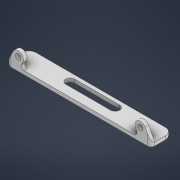
# Autodesk Inventor part: PCB Mount Support
Saved by Autodesk Inventor 2022.1 (Build 261234000, 234)
## iProperties
Created: 2022-01-06
Part Number: PCB Mount Support
Material: Generic
Document SubType Name: Modeling
Designer: Santiago Martínez
Mass: 1.78141 g
Surface Area: 23.5704 cm^2
Volume: 1.78141 cm^3
Density: 1 g/cm^3
Appearance: Default
Author: Santiago Martínez
Autodesk Inventor part; units mm, degrees
ref_plane "YZ Plane" through (0, 0, 0) normal (1, 0, 0) x (0, 1, 0)
ref_plane "XZ Plane" through (0, 0, 0) normal (0, 1, 0) x (-1, 0, 0)
ref_plane "XY Plane" through (0, 0, 0) normal (0, 0, 1) x (1, 0, 0)
sketch "Sketch1" plane through (0, 0, 0) normal (0, 1, 0) x (-1, 0, 0)
  line L0 (-27.5, -7.5) -> (-52.5, -7.5) construction
  line L1 (-27.5, -5) -> (-52.5, -5)
  line L2 (-52.5, -10) -> (-27.5, -10)
  arc A0 (-27.5, -10) -> (-27.5, -5) centre (-27.5, -7.5) ccw
  arc A1 (-52.5, -5) -> (-52.5, -10) centre (-52.5, -7.5) ccw
  line L3 (-4, -12) -> (-76, -12)
  line L4 (-80, -8) -> (-80, 0)
  line L5 (-80, 0) -> (0, 0)
  line L6 (0, 0) -> (0, -8)
  arc A2 (-4, -12) -> (0, -8) centre (-4, -8) ccw
  arc A3 (-80, -8) -> (-76, -12) centre (-76, -8) ccw
  point P0 (-40, -7.5)
  point P1 (-80, -12)
  point P2 (-40, -12)
  dimension "d0" = 25
  dimension "d1" = 5
  dimension "d2" = 80
  dimension "d3" = 12
  dimension "d5" = 4
  dimension "d6" = 2
  constraints: 16 end point, 8 point on circle, 8 tangent, 4 centre point, 3 parallel, 2 horizontal, 2 midpoint, 2 point on line, 1 coincident, 1 equal radius, 1 perpendicular, 1 vertical alignment
  measures "d0" distance of L0.start L0.end
  measures "d1" diameter of A1
  measures "d2" distance of L4.end L5.end
  measures "d3" distance of point (-80, -12) L4.end
  measures "d5" radius of A2
  measures "d6" distance between parallel lines of L2 L3
extrude "Extrusion1" add sketch "Sketch1" along normal blind 2
sketch "Sketch2" plane through (0, 0, 0) normal (0, 0, 1) x (1, 0, 0)
  circle A0 centre (6, 7) radius 1.5
  circle A1 centre (74, 7) radius 1.5
  line L0 (0, 0) -> (0, 2) projected
  line L1 (80, 0) -> (80, 2) projected
  line L2 (0, 2) -> (80, 2) projected
  line L3 (4, 2) -> (0, 2) projected
  line L4 (76, 2) -> (4, 2) projected
  line L5 (9.2479, 2) -> (12, 2)
  arc A2 (8.6585, 5.6098) -> (3.3415, 8.3902) centre (6, 7) ccw
  line L6 (0, 2) -> (3.3415, 8.3902)
  line L7 (7.9187, 4.1951) -> (8.6585, 5.6098)
  arc A3 (7.9187, 4.1951) -> (9.2479, 2) centre (9.2479, 3.5) ccw
  arc A4 (76.6585, 8.3902) -> (71.3415, 5.6098) centre (74, 7) ccw
  line L8 (80, 2) -> (76.6585, 8.3902)
  line L9 (71.3415, 5.6098) -> (72.0813, 4.1951)
  line L10 (70.7521, 2) -> (70.1315, 2)
  arc A5 (70.7521, 2) -> (72.0813, 4.1951) centre (70.7521, 3.5) ccw
  point P0 (6.7708, 2)
  point P1 (73.2292, 2)
  point P2 (9.2479, 2)
  dimension "d9" = 3
  dimension "d10" = 3
  dimension "d11" = 6
  dimension "d12" = 6
  dimension "d13" = 5
  dimension "d16" = 6
  dimension "d17" = 1.5
  dimension "d18" = 6
  dimension "d19" = 1.5
  constraints: 12 end point, 8 point on circle, 8 point on line, 8 tangent, 6 centre point, 2 coincident, 2 parallel, 1 collinear, 1 horizontal alignment
  measures "d9" diameter of A0
  measures "d10" diameter of A1
  measures "d11" distance from line of L0 A0.centre
  measures "d12" distance from line of A1.centre L1
  measures "d13" distance from line of L2 A0.centre
  measures "d16" diameter of A2
  measures "d17" radius of A3
  measures "d18" diameter of A4
  measures "d19" radius of A5
extrude "Extrusion2" add sketch "Sketch2" against normal blind 2
fillet "Fillet1" radius 2 2 edges at (0, 1, 0) (80, 1, 0)
equation "\"d10\" = d9"
equation "\"d12\" = d11"
equation "\"d18\" = d16"
equation "\"d19\" = d17"
body "Solid1"
